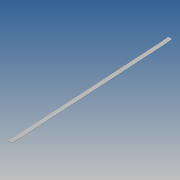
# Autodesk Inventor part: 2p6fs2
Saved by Autodesk Inventor 2014 SP1 (Build 180222100, 222)
## iProperties
Company: HERA Project
Created: 2013-12-11
Part Number: 2p6fs2
Material: Steel
Document SubType Name: Sheet Metal
Designer: David DeBoer
Mass: 1118.84 g
Surface Area: 1199.54 cm^2
Volume: 142.527 cm^3
Density: 7.85 g/cm^3
Description: second furring strip
Appearance: Steel
Sheet Metal Rule: Default
Author: David DeBoer
Autodesk Inventor part; units mm, degrees
ref_plane "YZ Plane" through (0, 0, 0) normal (1, 0, 0) x (0, 1, 0)
ref_plane "XZ Plane" through (0, 0, 0) normal (0, 1, 0) x (-1, 0, 0)
ref_plane "XY Plane" through (0, 0, 0) normal (0, 0, 1) x (1, 0, 0)
sketch "Sketch1" plane through (0, 0, 0) normal (0, 0, 1) x (1, 0, 0)
  line L0 (0, 0) -> (38.1, 0)
  line L1 (38.1, 0) -> (38.1, 3.048)
  line L2 (38.1, 3.048) -> (0, 3.048)
  line L3 (0, 3.048) -> (0, 0)
  dimension "d0" = 38.1
  dimension "d1" = 3.048
  constraints: 8 end point, 2 parallel, 1 horizontal, 1 perpendicular
  measures "d0" distance of L0.start L0.end
  measures "d1" distance of L2.end L0.start
extrude "Extrusion1" add sketch "Sketch1" along normal blind 1615
sketch "Sketch2" plane through (0, 3.048, 0) normal (0, 1, 0) x (1, 0, 0)
  line L0 (38.1, 0) -> (0, 0) projected
  circle A0 centre (19.05, -20) radius 2.2451
  dimension "d4" = 20
  constraints: 1 centre point
  measures "d4" distance from line of A0.centre L0
hole "Hole1" at (19.05, 3.048, 20) direction (0, -1, 0) diameter 3.175 end through all
sketch "Sketch3" plane through (0, 3.048, 0) normal (0, 1, 0) x (1, 0, 0)
  line L0 (38.1, -1615) -> (0, -1615) projected
  circle A0 centre (19.05, -1595) radius 2.2451
  dimension "d12" = 20
  constraints: 1 centre point
  measures "d12" distance from line of L0 A0.centre
hole "Hole2" at (19.05, 3.048, 1595) direction (0, -1, 0) diameter 3.175 end through all
sketch "Sketch4" plane through (0, 3.048, 0) normal (0, 1, 0) x (1, 0, 0)
  circle A0 centre (19.05, -1595) radius 1.5875 projected
  line L0 (0, 0) -> (0, -1615) projected
  line L1 (38.1, 0) -> (38.1, -1615) projected
  line L2 (0, -1535) -> (38.1, -1535)
  line L3 (0, -1535) -> (38.1, -1535)
  line L4 (0, -1535) -> (56.1267, -1535) construction
  dimension "d20" = 60
  dimension "d21" = 0
  constraints: 6 end point, 3 point on line, 1 horizontal, 1 perpendicular
  measures "d20" distance from line of L2 A0.centre
  measures "d21" distance between parallel lines of L4 L3
fold "Fold1" angle 3.5 bend radius 3.048 thickness 3.048 k factor 0.44 line from (0, 3.048, 1535) to (38.1, 3.048, 1535) line at bend centre moving side (0, 0, -1) folds toward (0, 1, 0)
sketch "Sketch5" plane through (0, 96.755, 2.9449) normal (0, 0.9981348, 0.0610485) x (1, 0, 0)
  line L0 (38.1, 0) -> (38.1, -1534.8659) projected
  line L1 (0, 0) -> (0, -1534.8659) projected
  circle A0 centre (19.05, -20) radius 1.5875 projected
  line L2 (0, -80) -> (38.1, -80)
  line L3 (0, -80) -> (38.1, -80)
  line L4 (0, -80) -> (69.3838, -80) construction
  dimension "d28" = 60
  dimension "d29" = 0
  constraints: 6 end point, 3 point on line, 1 horizontal, 1 perpendicular
  measures "d28" distance from line of L2 A0.centre
  measures "d29" distance between parallel lines of L3 L4
fold "Fold2" angle 3.5 bend radius 3.048 thickness 3.048 k factor 0.44 line from (0, 91.8711, 82.7957) to (38.1, 91.8711, 82.7957) line at bend centre moving side (0, 0.0610485, -0.9981348) folds toward (0, 0.9981348, 0.0610485)
equation "\"d1\" = Thickness"
equation "\"d22\" = BendReliefWidth"
equation "\"d23\" = BendReliefDepth"
equation "\"d24\" = MinimumRemnant"
equation "\"d25\" = BendRadius"
equation "\"d26\" = foldAngle"
equation "\"d27\" = BendRadius"
equation "\"d30\" = BendReliefWidth"
equation "\"d31\" = BendReliefDepth"
equation "\"d32\" = MinimumRemnant"
equation "\"d33\" = BendRadius"
equation "\"d34\" = foldAngle"
equation "\"d35\" = BendRadius"
equation "\"BendRadius\" = Thickness"
equation "\"BendReliefWidth\" = Thickness"
equation "\"BendReliefDepth\" = 0.5 * Thickness"
equation "\"CornerReliefSize\" = 4 * Thickness"
equation "\"MinimumRemnant\" = 2 * Thickness"
equation "\"TransitionRadius\" = BendRadius"
equation "\"JacobiRadiusSize\" = Thickness"
equation "\"GapSize\" = Thickness"
equation "\"foldAngle\" = 3.5deg"
equation "\"Thickness\" = 3.048"
body "Solid1"
